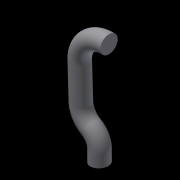
# Autodesk Inventor part: CO2FeedPipe
Saved by Autodesk Inventor 2020.4 (Build 244396010, 396A)
## iProperties
Created: 2022-09-17
Part Number: CO2FeedPipe
Material: Generic
Document SubType Name: Modeling
Designer: Val
Density: 1 g/cm^3
Appearance: Default
Author: Val
Autodesk Inventor part; units mm, degrees
ref_plane "YZ Plane" through (0, 0, 0) normal (1, 0, 0) x (0, 1, 0)
ref_plane "XZ Plane" through (0, 0, 0) normal (0, 1, 0) x (-1, 0, 0)
ref_plane "XY Plane" through (0, 0, 0) normal (0, 0, 1) x (1, 0, 0)
sketch "Sketch2" plane through (0, 0, 0) normal (1, 0, 0) x (0, 1, 0)
  circle A0 centre (332.9239, 1.3141) radius 25.4
  point P0 (0, 0)
  point P1 (332.9239, 0)
  dimension "d7" = 50.8
  constraints: 1 centre point
  measures "d7" diameter of A0
sketch "Sketch1" plane through (0, 0, 0) normal (0, 0, 1) x (1, 0, 0)
  arc A0 (0, 332.9239) -> (-57.0054, 253.3863) centre (23.3842, 255.9672) ccw
  arc A1 (-53.7436, 151.7863) -> (-33.7941, 79.6763) centre (104.9754, 156.8819) ccw
  line L0 (-57.0054, 253.3863) -> (-53.7436, 151.7863)
  line L1 (0, -68.5181) -> (0, 411.1086) projected
  arc A2 (-27.6628, 56.0446) -> (-33.7941, 79.6763) centre (-76.2696, 56.0446) ccw
  line L2 (-27.6628, 56.0446) -> (-27.6628, 6.4982)
  point P0 (0, 0)
  dimension "d0" = 80.4311
  dimension "d2" = 101.6
  dimension "d5" = 332.9239
  constraints: 6 point on circle, 4 end point, 4 tangent, 3 centre point, 1 point on line, 1 vertical
  measures "d0" radius of A0
  measures "d2" vertical distance of L0.start L0.end
  measures "d5" distance of point (0, 0) A0.start
sweep "Sweep1" add profiles "Sketch2" path "Sketch1" path curves A0 L0 A1 A2 L2
body "Solid1"
